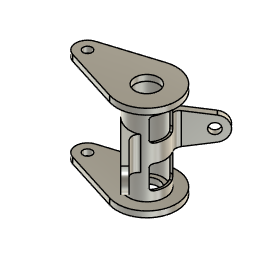
exercise09 (Autodesk Fusion 360 design; units mm, degrees)
Autodesk Fusion 360 part; units mm, degrees
sketch "草图1" plane through (0, 0, 0) normal (0, 0, 1) x (1, 0, 0)
  circle A0 centre (0, 0) radius 0.69
  circle A1 centre (0, 0) radius 0.78
  circle A2 centre (0, 0) radius 0.5
  circle A3 centre (-2.5, 0) radius 0.19
  line L0 (-2.65, 0.477) -> (-0.375, 1.1924)
  line L1 (-2.65, -0.477) -> (-0.375, -1.1924)
  arc A4 (-2.65, 0.477) -> (-2.65, -0.477) centre (-2.5, 0) ccw
  line L2 (-2.5, 0) -> (-2.31, 0)
  arc A5 (-0.375, -1.1924) -> (-0.375, 1.1924) centre (0, 0) ccw
  dimension "d1" = 1.38
  dimension "d2" = 1.56
  dimension "d3" = 1
  dimension "d4" = 2.5
  dimension "d5" = 0.38
  dimension "d6" = 1
  dimension "d7" = 2.5
  constraint coincident A0.centre A1.centre
  constraint concentric A1 A2
  constraint concentric A3 A4
  constraint tangent L0 A4
  constraint tangent L1 A4
  constraint tangent L1 A5
  constraint tangent L0 A5
  constraint coincident A3.centre A4.centre
  constraint horizontal L2
  constraint coincident A3 L2.end
  measures "d1" diameter of A0
  measures "d2" diameter of A1
  measures "d3" diameter of A2
  measures "d4" diameter of A5
  measures "d5" diameter of A3
  measures "d6" diameter of A4
  measures "d7" distance of A0.centre A3.centre
extrude "拉伸1" add sketch "草图1" against normal blind 0.25 contours A0 | A1 | L0 L1 A4 A5 makes body 1
extrude "拉伸2" add sketch "草图1" along normal blind 3.5 separate body contours A1 makes body 2
copy_body "复制和粘贴实体1" bodies 1 makes body 3
move_body "移动1" bodies 3 to x (1, 0, 0) y (0, 1, 0) z (0, 0, 1) at (0, 0, 3.75)
sketch "草图2" plane through (0, 0, 0) normal (1, 0, 0) x (0, 1, 0)
  line L0 (-0.375, 3.12) -> (0.375, 3.12)
  line L1 (0.5, 2.995) -> (0.5, 2.245)
  line L2 (0.375, 2.12) -> (-0.375, 2.12)
  line L3 (-0.5, 2.245) -> (-0.5, 2.995)
  line L4 (-0.375, 1.38) -> (0.375, 1.38)
  line L5 (0.5, 1.255) -> (0.5, 0.505)
  line L6 (0.375, 0.38) -> (-0.375, 0.38)
  line L7 (-0.5, 0.505) -> (-0.5, 1.255)
  arc A0 (-0.375, 3.12) -> (-0.5, 2.995) centre (-0.375, 2.995) ccw
  arc A1 (0.5, 2.995) -> (0.375, 3.12) centre (0.375, 2.995) ccw
  arc A2 (0.375, 0.38) -> (0.5, 0.505) centre (0.375, 0.505) ccw
  arc A3 (-0.5, 0.505) -> (-0.375, 0.38) centre (-0.375, 0.505) ccw
  arc A4 (-0.375, 1.38) -> (-0.5, 1.255) centre (-0.375, 1.255) ccw
  arc A5 (0.5, 1.255) -> (0.375, 1.38) centre (0.375, 1.255) ccw
  arc A6 (0.375, 2.12) -> (0.5, 2.245) centre (0.375, 2.245) ccw
  arc A7 (-0.5, 2.245) -> (-0.375, 2.12) centre (-0.375, 2.245) ccw
  line L8 (0, 4) -> (0, -0.5512) construction
  dimension "d12" = 0.125
  dimension "d13" = 1
  dimension "d14" = 2.74
  dimension "d15" = 0.38
  constraint horizontal L0
  constraint vertical L1
  constraint horizontal L2
  constraint vertical L3
  constraint horizontal L4
  constraint vertical L5
  constraint horizontal L6
  constraint vertical L7
  constraint tangent L0 A0
  constraint tangent L3 A0
  constraint tangent L0 A1
  constraint tangent L1 A1
  constraint equal A0 A1
  constraint tangent L5 A2
  constraint tangent L6 A2
  constraint equal A0 A2
  constraint tangent L6 A3
  constraint tangent L7 A3
  constraint equal A0 A3
  constraint tangent L4 A4
  constraint tangent L7 A4
  constraint equal A0 A4
  constraint tangent L4 A5
  constraint tangent L5 A5
  constraint equal A0 A5
  constraint tangent L1 A6
  constraint tangent L2 A6
  constraint equal A0 A6
  constraint tangent L2 A7
  constraint tangent L3 A7
  constraint equal A0 A7
  constraint equal L0 L4
  constraint equal L0 L3
  constraint equal L4 L7
  constraint parallel L1 L8
  constraint symmetric L1 L3 L8
  constraint symmetric L5 L7 L8
  measures "d12" radius of A0
  measures "d13" distance of L0 L2
  measures "d14" distance of L0 L6
  measures "d15" distance of origin L6
extrude "拉伸3" cut sketch "草图2" along normal blind 0.78 contours L0 L1 L2 L3 A0 A1 A6 A7 bodies 2
extrude "拉伸4" cut sketch "草图2" along normal blind 0.78 contours L4 L5 L6 L7 A2 A3 A4 A5 bodies 2
ref_plane "工作平面1" through (0, 0, 1.75) normal (0, 0, 1) x (1, 0, 0)
sketch "草图3" plane through (0, 0, 1.75) normal (0, 0, 1) x (1, 0, 0)
  circle A0 centre (0, 0) radius 0.78
  circle A1 centre (0, 0) radius 0.69
  line L0 (2.6, 0) -> (-1.7605, 0) construction
  line L1 (1.2375, 2.3406) -> (1.4143, 2.1638)
  line L2 (1.4143, 2.1638) -> (0.3536, 1.1032)
  line L3 (0.3536, 1.1032) -> (0.1768, 1.2799)
  line L4 (0.1768, 1.2799) -> (1.2375, 2.3406)
  line L5 (0.3536, -1.1032) -> (0.1768, -1.2799)
  line L6 (0.1768, -1.2799) -> (1.2375, -2.3406)
  line L7 (1.2375, -2.3406) -> (1.4143, -2.1638)
  line L8 (1.4143, -2.1638) -> (0.3536, -1.1032)
  arc A2 (0.3536, 1.1032) -> (0.4059, 0.6661) centre (0.5516, 0.9052) ccw
  arc A3 (0.4059, -0.6661) -> (0.3536, -1.1032) centre (0.5516, -0.9052) ccw
  line L9 (0.1768, 1.2799) -> (-0.5515, 0.5515)
  line L10 (0.1768, -1.2799) -> (-0.5515, -0.5515)
  dimension "d21" = 1.56
  dimension "d22" = 1.38
  dimension "d23" = 0.25
  dimension "d24" = 45
  dimension "d25" = 1.5
  dimension "d26" = 0.28
  constraint coincident A0.centre A1.centre
  constraint horizontal L0
  constraint perpendicular L1 L2
  constraint parallel L1 L3
  constraint parallel L2 L4
  constraint perpendicular L5 L6
  constraint parallel L5 L7
  constraint parallel L6 L8
  constraint symmetric L0 L2.end L5.start
  constraint symmetric L0 L1.start L6.end
  constraint symmetric L0 L1.end L7.end
  constraint coincident A0 A2.end
  constraint tangent L8 A3
  constraint coincident A0 A3.start
  constraint tangent A0 A3
  constraint tangent A0 A2
  constraint equal A2 A3
  constraint tangent L2 A2
  constraint coincident A0 L9.end
  constraint tangent A0 L9
  constraint coincident A0 L10.end
  constraint tangent A0 L10
  constraint parallel L4 L9
  measures "d21" diameter of A0
  measures "d22" diameter of A1
  measures "d23" distance of L1.start L1.end
  measures "d24" angle of L0 L2
  measures "d25" distance of L1.start L3.end
  measures "d26" radius of A2
extrude "拉伸5" add sketch "草图3" along normal mid plane 1.62 separate body makes body 4
sketch "草图4" plane through (-0.5515, -0.5515, 0) normal (-0.707107, -0.707107, 0) x (0.707107, -0.707107, 0)
  line L0 (2.5301, 0.94) -> (2.5301, 2.56)
  line L1 (2.5301, 2.56) -> (0, 2.56)
  line L2 (0, 2.56) -> (0, 0.94)
  line L3 (0, 0.94) -> (2.5301, 0.94)
  circle A0 centre (2.0301, 1.75) radius 0.22
  circle A1 centre (2.0301, 1.75) radius 0.5
  line L4 (0, 2.56) -> (2.1042, 2.2445)
  line L5 (0, 0.94) -> (2.1042, 1.2555)
  line L6 (0, 2.56) -> (0, 0.94)
  dimension "d29" = 1
  dimension "d30" = 0.44
  dimension "d31" = 0.81
  constraint concentric A0 A1
  constraint coincident L1.end L2.start
  constraint coincident A1 L4.end
  constraint tangent A1 L4
  constraint coincident L2.end L3.start
  constraint coincident A1 L5.end
  constraint tangent A1 L5
  constraint tangent L0 A1
  measures "d29" diameter of A1
  measures "d30" diameter of A0
  measures "d31" distance of L1 A0.centre
extrude "拉伸6" cut sketch "草图4" against normal blind 1.2 contours L0 L3 A1 L5 | L0 L1 A1 L4 | A0 bodies 4
sketch "草图5" plane through (-0.5515, 0.5515, 0) normal (-0.707107, 0.707107, 0) x (-0.707107, -0.707107, 0)
  line L0 (0, 0.94) -> (0, 2.56)
  line L1 (0, 2.56) -> (-2.5301, 2.56)
  line L2 (-2.5301, 2.56) -> (-2.5301, 0.94)
  line L3 (-2.5301, 0.94) -> (0, 0.94)
  circle A0 centre (-2.0301, 1.75) radius 0.5
  circle A1 centre (-2.0301, 1.75) radius 0.22
  line L4 (0, 2.56) -> (0, 0.94)
  line L5 (0, 0.94) -> (-2.1042, 1.2555)
  line L6 (0, 2.56) -> (-2.1042, 2.2445)
  dimension "d34" = 1
  dimension "d35" = 0.44
  dimension "d36" = 0.81
  constraint concentric A0 A1
  constraint coincident L0.end L1.start
  constraint coincident L0.start L3.end
  constraint coincident A0 L5.end
  constraint tangent A0 L5
  constraint coincident A0 L6.end
  constraint tangent A0 L6
  constraint tangent L2 A0
  measures "d34" diameter of A0
  measures "d35" diameter of A1
  measures "d36" vertical distance of L1.end A0.centre
extrude "拉伸7" cut sketch "草图5" against normal blind 2.6 contours L2 L3 A0 L5 | L1 L2 A0 L6 | A1 bodies 4
extrude "拉伸8" cut sketch "草图2" along normal blind 0.599 bodies 4
extrude "拉伸9" cut sketch "草图2" along normal blind 5.4 bodies 4
combine "合并1" operation add target body 1 tool bodies 2 3 4
equation "d14 = 3.5 mm - 0.38 mm - 0.38 mm"
